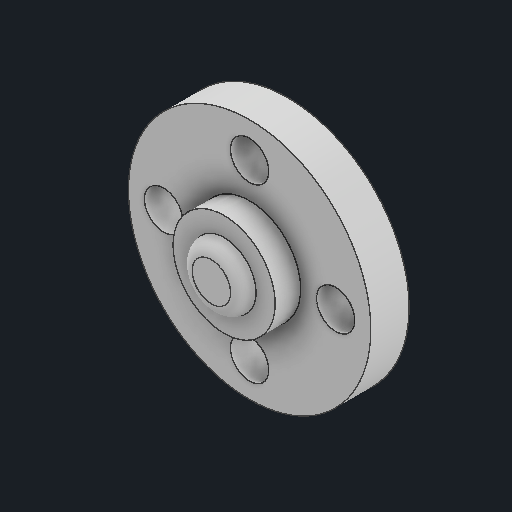
# Autodesk Inventor part: FeeTechSTS3025BL-Flange
Saved by Autodesk Inventor 2025.2 (Build 292293000, 293)
## iProperties
Created: 2025-07-26
Part Number: FeeTechSTS3025BL-Flange
Material: Generic
Document SubType Name: Modeling
Designer: valer
Density: 1 g/cm^3
Appearance: Default
Author: valer
Autodesk Inventor part; units mm, degrees
ref_plane "YZ Plane" through (0, 0, 0) normal (1, 0, 0) x (0, 1, 0)
ref_plane "XZ Plane" through (0, 0, 0) normal (0, 1, 0) x (-1, 0, 0)
ref_plane "XY Plane" through (0, 0, 0) normal (0, 0, 1) x (1, 0, 0)
sketch "Sketch1" plane through (0, 0, 0) normal (0, 0, 1) x (1, 0, 0)
  circle A0 centre (0, 0) radius 9.5
  dimension "d0" = 19
  constraints: 1 centre point, 1 coincident
  measures "d0" diameter of A0
extrude "Extrusion1" add sketch "Sketch1" along normal blind 3
sketch "Sketch2" plane through (0, 0, 3) normal (0, 0, 1) x (1, 0, 0)
  circle A0 centre (0, 0) radius 9.5 projected
  circle A1 centre (0, 0) radius 4
  dimension "d3" = 8
  constraints: 1 centre point, 1 coincident
  measures "d3" diameter of A1
extrude "Extrusion2" add sketch "Sketch2" along normal blind 2 contours A1
sketch "Sketch3" plane through (0, 0, 5) normal (0, 0, 1) x (1, 0, 0)
  circle A0 centre (0, 0) radius 4 projected
  circle A1 centre (0, 0) radius 2.5
  dimension "d6" = 5
  constraints: 1 centre point, 1 coincident
  measures "d6" diameter of A1
extrude "Extrusion3" add sketch "Sketch3" along normal blind 1 contours A1
fillet "Fillet1" radius 1 1 edges at (-2.5, 0, 6)
sketch "Sketch4" plane through (0, 0, 3) normal (0, 0, 1) x (1, 0, 0)
  circle A0 centre (0, 0) radius 4 projected
  line L0 (0, 4) -> (0, 9.5)
  circle A1 centre (0, 0) radius 9.5 projected
  line L1 (-9.5, 0) -> (-4, 0)
  line L2 (-13.3, 0) -> (13.3, 0) construction
  line L3 (0, -13.3) -> (0, 13.3) construction
  circle A2 centre (0, 6.75) radius 1.5
  circle A3 centre (0, -6.75) radius 1.5
  circle A4 centre (-6.75, 0) radius 1.5
  circle A5 centre (6.75, 0) radius 1.5
  dimension "d10" = 3
  constraints: 4 centre point, 4 end point, 4 point on circle, 2 coincident, 2 collinear, 2 midpoint, 2 symmetric about line, 1 equal radius, 1 horizontal, 1 vertical, 2 other
  measures "d10" diameter of A2
extrude "Extrusion4" cut sketch "Sketch4" against normal through all contours A2 L0 | L0 A2 | A4 L1 | L1 A4 | A3 | A5
sketch "Sketch5" plane through (0, 0, 0) normal (0, 0, -1) x (-1, 0, 0)
  circle A0 centre (0, 0) radius 2.5 projected
extrude "Extrusion5" add sketch "Sketch5" along normal blind 1
body "Solid1"
